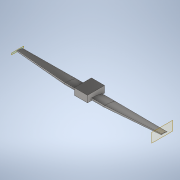
# Autodesk Inventor part: Glider Box
Saved by Autodesk Inventor 2021 (Build 250183000, 183)
## iProperties
Created: 2021-01-25
Part Number: Glider Box
Material: Generic
Document SubType Name: Modeling
Designer: david
Density: 1 g/cm^3
Appearance: Diamond Plate
Author: david
Autodesk Inventor part; units mm, degrees
ref_plane "YZ Plane" through (0, 0, 0) normal (1, 0, 0) x (0, 1, 0)
ref_plane "XZ Plane" through (0, 0, 0) normal (0, 1, 0) x (-1, 0, 0)
ref_plane "XY Plane" through (0, 0, 0) normal (0, 0, 1) x (1, 0, 0)
sketch "Sketch1" plane through (0, 0, 0) normal (0, 1, 0) x (-1, 0, 0)
  line L0 (115.4545, -16.1636) -> (-138.5455, -16.1636)
  line L1 (-138.5455, -16.1636) -> (-138.5455, -346.3636)
  line L2 (-138.5455, -346.3636) -> (115.4545, -346.3636)
  line L3 (115.4545, -346.3636) -> (115.4545, -16.1636)
  point P0 (0, 0)
  dimension "d0" = 254
  dimension "d1" = 330.2
  constraints: 8 end point, 2 parallel, 1 horizontal, 1 perpendicular
  measures "d0" distance between parallel lines of L1 L3
  measures "d1" distance of L2.end L0.start
extrude "Extrusion1" add sketch "Sketch1" along normal blind 127
sketch "Sketch2" plane through (138.5455, 0, -16.1636) normal (1, 0, 0) x (0, 0, -1)
  arc A0 (76.2, 44.45) -> (63.5, 25.4) centre (81.0618, 27.4505) ccw
  line L0 (76.2, 44.45) -> (177.2082, 44.45) construction
  line L1 (177.2082, 44.45) -> (279.4, 15.24) construction
  spline S0 degree 2 poles (76.2, 44.45) (177.2082, 44.45) (279.4, 15.24) knots 1 1 1 2 2 2
  line L2 (63.5, 25.4) -> (224.9578, 24.13) construction
  line L3 (224.9578, 24.13) -> (279.4, 15.24) construction
  spline S1 degree 2 poles (63.5, 25.4) (224.9578, 24.13) (279.4, 15.24) knots 1 1 1 2 2 2
  line L4 (0, 0) -> (330.2, 0) projected
  line L5 (0, 127) -> (330.2, 127) projected
  line L6 (0, 0) -> (0, 127) projected
  line L7 (330.2, 0) -> (330.2, 127) projected
  point P0 (-16.1636, 0)
  dimension "d4" = 25.4
  dimension "d5" = 15.24
  dimension "d6" = 24.13
  dimension "d7" = 82.55
  dimension "d8" = 82.55
  dimension "d9" = 63.5
  dimension "d10" = 76.2
  dimension "d11" = 50.8
  dimension "d12" = 101.0082
  dimension "d13" = 102.1918
  constraints: 2 point on circle, 1 centre point, 1 horizontal, 6 other
  measures "d4" distance from line of L4 L2.start
  measures "d5" distance from line of L4 L1.end
  measures "d6" distance from line of L4 L2.end
  measures "d7" distance from line of L5 L0.start
  measures "d8" distance from line of L5 L0.end
  measures "d9" distance from line of L6 L2.start
  measures "d10" distance from line of L6 L0.start
  measures "d11" distance from line of L1.end L7
  measures "d12" distance of L0.start L0.end
  measures "d13" horizontal distance of L0.end L1.end
extrude "Extrusion2" add sketch "Sketch2" along normal blind 254 and the other way blind 508 contours S0 S1 A0
ref_plane "Work Plane1" through (1408.5455, 0, -16.1636) normal (1, 0, 0) x (0, 0, -1)
sketch "Sketch5" plane through (1408.5455, 0, -16.1636) normal (1, 0, 0) x (0, 0, -1)
  arc A0 (76.2, 44.45) -> (63.5, 25.4) centre (81.0618, 27.4505) ccw projected
  spline S0 degree 2 poles (154.1033, 24.5678) (240.1651, 22.1028) (269.0908, 16.7605) knots 1 1 1 2 2 2
  spline S1 degree 2 poles (269.0908, 16.7605) (214.934, 33.4644) (161.0849, 34.5831) knots 1 1 1 2 2 2
  arc A1 (161.0849, 34.5831) -> (154.1033, 24.5678) centre (163.4885, 25.4665) ccw
  point P0 (-16.1636, 0)
  constraints: 2 point on circle, 1 centre point, 8 other
loft "Loft1" add profiles "Sketch5" section 1 edges at (392.5455, 22.225, -214.3675) (392.5455, 37.1475, -193.6678) (392.5455, 37.2582, -82.5139)
ref_plane "Work Plane3" through (-1385.4545, 0, -16.1636) normal (-1, 0, 0) x (0, 0, 1)
sketch "Sketch7" plane through (-1385.4545, 0, -16.1636) normal (-1, 0, 0) x (0, 0, 1)
  spline S0 degree 2 poles (-269.0908, 16.7605) (-240.1651, 22.1028) (-154.1033, 24.5678) knots 0 0 0 1 1 1 projected
  spline S1 degree 2 poles (-161.0849, 34.5831) (-214.934, 33.4644) (-269.0908, 16.7605) knots 0 0 0 1 1 1 projected
  arc A0 (-154.1033, 24.5678) -> (-161.0849, 34.5831) centre (-163.4885, 25.4665) ccw projected
  point P0 (16.1636, 0)
  constraints: 2 other
loft "Loft2" add profiles "Sketch7" section 2 edges at (-369.4545, 22.225, -214.3675) (-369.4545, 37.2582, -82.5139) (-369.4545, 37.1475, -193.6678)
body "Solid1"
